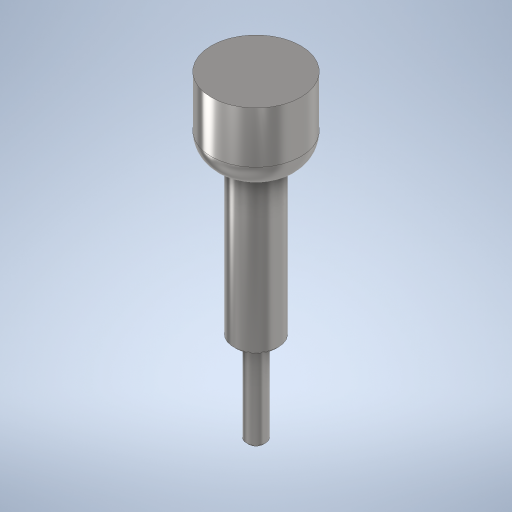
# Autodesk Inventor part: screwdriver
Saved by Autodesk Inventor 2024.3 (Build 283343000, 343)
## iProperties
Created: 2025-07-30
Part Number: screwdriver
Material: Acciaio inossidabile
Document SubType Name: Modeling
Designer: chris
Density: 8 g/cm^3
Appearance: Semilucidato
Author: chris
Autodesk Inventor part; units mm, degrees
ref_plane "YZ Plane" through (0, 0, 0) normal (1, 0, 0) x (0, 1, 0)
ref_plane "XZ Plane" through (0, 0, 0) normal (0, 1, 0) x (-1, 0, 0)
ref_plane "XY Plane" through (0, 0, 0) normal (0, 0, 1) x (1, 0, 0)
sketch "Schizzo1" plane through (0, 0, 0) normal (0, 0, 1) x (1, 0, 0)
  circle A0 centre (0, 0) radius 0.035
  dimension "d0" = 0.07
  constraints: 1 centre point, 1 coincident
  measures "d0" diameter of A0
extrude "Estrusione1" add sketch "Schizzo1" along normal blind 0.06
sketch "Schizzo6" plane through (0, 0, 0.06) normal (0, 0, 1) x (1, 0, 0)
  circle A0 centre (0, 0) radius 0.0175
  dimension "d20" = 0.035
  constraints: 1 centre point, 1 coincident
  measures "d20" diameter of A0
extrude "Estrusione5" add sketch "Schizzo6" along normal blind 0.19
sketch "Schizzo7" plane through (0, 0, 0.25) normal (0, 0, 1) x (1, 0, 0)
  circle A0 centre (0, 0) radius 0.0175 projected
  circle A1 centre (0, 0) radius 0.0075
  dimension "d23" = 0.015
  constraints: 1 centre point, 1 coincident
  measures "d23" diameter of A1
extrude "Estrusione6" cut sketch "Schizzo7" against normal blind 0.07
fillet "Raccordo4" radius 0.02 1 edges at (-0.035, 0, 0.06)
chamfer "Smusso2" distance 0.002 angle 45 2 edges at (-0.0175, 0, 0.18) (-0.0075, 0, 0.25)
